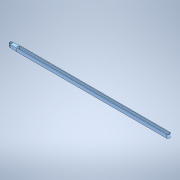
# Autodesk Inventor part: arm
Saved by Autodesk Inventor 2022 (Build 260153000, 153)
## iProperties
Created: 2022-10-28
Part Number: arm
Material: Generic
Document SubType Name: Modeling
Designer: matia
Density: 1 g/cm^3
Appearance: Default
Author: matia
Autodesk Inventor part; units mm, degrees
ref_plane "YZ Plane" through (0, 0, 0) normal (1, 0, 0) x (0, 1, 0)
ref_plane "XZ Plane" through (0, 0, 0) normal (0, 1, 0) x (-1, 0, 0)
ref_plane "XY Plane" through (0, 0, 0) normal (0, 0, 1) x (1, 0, 0)
sketch "Sketch1" plane through (0, 0, 0) normal (0, 1, 0) x (-1, 0, 0)
  circle A0 centre (0, 0) radius 4.445
  line L0 (4.445, 0) -> (5.715, 0)
  line L1 (0, 4.445) -> (0, 5.715)
  line L2 (0, -4.445) -> (0, -5.715)
  line L3 (0, -5.715) -> (2.54, -5.715)
  line L4 (2.54, -5.715) -> (-2.54, -5.715)
  line L5 (0, 5.715) -> (2.54, 5.715)
  line L6 (2.54, 5.715) -> (-2.54, 5.715)
  line L7 (5.715, 0) -> (5.461, 0)
  line L8 (5.715, 0) -> (5.715, 2.54)
  line L9 (5.715, 2.54) -> (5.715, -2.54)
  line L10 (5.715, -2.54) -> (5.715, 2.54)
  line L11 (2.54, 5.715) -> (5.715, 2.54)
  line L12 (5.715, -2.54) -> (2.54, -5.715)
  line L13 (20.955, 0) -> (-4.445, 0)
  arc A1 (-29.845, -6.223) -> (-29.845, 4.445) centre (-29.845, -0.889) ccw
  line L14 (-29.845, -6.223) -> (-29.845, -8.763)
  line L15 (-29.845, 4.445) -> (-29.845, 6.985)
  line L16 (-29.845, 6.985) -> (-2.54, 5.715)
  line L17 (-2.54, -5.715) -> (-29.845, -8.763)
  line L18 (-29.845, 6.985) -> (-639.445, 6.985)
  line L19 (-29.845, -8.763) -> (-639.445, -8.763)
  line L20 (-29.845, 4.445) -> (-639.445, 4.445)
  line L21 (-29.845, -6.223) -> (-90.805, -6.223)
  arc A2 (-639.445, 6.985) -> (-639.445, -8.763) centre (-639.445, -0.889) ccw
  line L22 (-29.845, -6.223) -> (-639.445, -6.223)
  arc A3 (-639.445, 4.445) -> (-639.445, -6.223) centre (-639.445, -0.889) ccw
  dimension "d0" = 8.89
  dimension "d1" = 1.27
  dimension "d2" = 1.27
  dimension "d3" = 1.27
  dimension "d4" = 2.54
  dimension "d5" = 5.08
  dimension "d6" = 2.54
  dimension "d7" = 5.08
  dimension "d8" = 0.254
  dimension "d9" = 2.54
  dimension "d10" = 5.08
  dimension "d11" = 25.4
  dimension "d12" = 10.668
  dimension "d13" = 2.54
  dimension "d14" = 2.54
  dimension "d15" = 609.6
  dimension "d16" = 609.6
  dimension "d17" = 609.6
  dimension "d18" = 60.96
  dimension "d19" = 609.6
  constraints: 46 end point, 9 point on circle, 6 horizontal, 6 point on line, 5 vertical, 4 centre point, 3 perpendicular, 2 coincident, 1 collinear
  measures "d0" diameter of A0
  measures "d1" distance of L0.start L0.end
  measures "d2" distance of L1.start L1.end
  measures "d3" distance of L2.start L2.end
  measures "d4" distance of L2.end L3.end
  measures "d5" distance of L3.end L4.end
  measures "d6" distance of L1.end L5.end
  measures "d7" distance of L5.end L6.end
  measures "d8" distance of L0.end L7.end
  measures "d9" distance of L0.end L8.end
  measures "d10" distance of L8.end L9.end
  measures "d11" distance of L13.start L13.end
  measures "d12" diameter of A1
  measures "d13" distance of L14.start L14.end
  measures "d14" distance of L15.start L15.end
  measures "d15" distance of L18.end L15.end
  measures "d16" distance of L19.end L14.end
  measures "d17" distance of L15.start L20.end
  measures "d18" distance of L14.start L21.end
  measures "d19" distance of L14.start L22.end
extrude "Extrusion1" add sketch "Sketch1" along normal blind 12.7 contours L0 L9 L12 L3 L2 A0 | A0 L1 L5 L11 L8 L0 | A0 L2 L4 L17 L14 A1 L15 L16 L6 L1 | L15 L20 A3 L22 L21 L14 L19 A2 L18
sketch "Sketch2" plane through (-2.54, 0, 5.715) normal (0, 0, 1) x (1, 0, 0)
  line L0 (2.54, 0) -> (2.54, 12.7)
  line L1 (0, 12.7) -> (5.08, 12.7) projected
  circle A0 centre (2.54, 6.35) radius 1.5875
  dimension "d22" = 3.175
  constraints: 2 end point, 2 midpoint, 1 centre point
  measures "d22" diameter of A0
hole "Hole1" at (0, 6.35, 5.715) direction (0, 0, -1) diameter 2.4867 end through all thread size "5-40 UNC" class "2B" standard "ANSI Unified Screw Threads"
body "Solid1"
